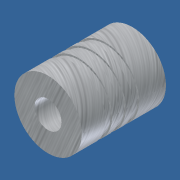
# Autodesk Inventor part: 25772-02
Saved by Autodesk Inventor 2014 (Build 180170000, 170)
## iProperties
Category: stocked
Created: 2011-08-08
Part Number: 25772-02
Document SubType Name: Modeling
Designer: ERF
Density: 2.71 g/cm^3
Description: Z-Axis Flexible Coupler 5mm - 8mm bore
Vendor: Robot Electron
Mass: 18.6653 g
Surface Area: 28.0725 cm^2
Volume: 6.88757 cm^3
Material: Aluminum 6061
Stock Number: ebay
Project: Shapeoko
Appearance: Aluminum (Machined)
Catalog Web Link: http://www.ebay.com/itm/5x5-5x8-5x10-6-35x8-6-35x12-8x8-6x14mm-CNC-Motor-Jaw-Shaft-Coupler-/330796927548
Authority: PER ALLEN @ ROBOT ELECTRON 9-12-13
Title: Flexible Coupler
Author: ERF
Subject: Motion
Comments: Fusion
Autodesk Inventor part; units mm, degrees
ref_plane "YZ Plane" through (0, 0, 0) normal (1, 0, 0) x (0, 1, 0)
ref_plane "XZ Plane" through (0, 0, 0) normal (0, 1, 0) x (-1, 0, 0)
ref_plane "XY Plane" through (0, 0, 0) normal (0, 0, 1) x (1, 0, 0)
sketch "Sketch1" plane through (0, 0, 0) normal (0, 0, 1) x (1, 0, 0)
  circle A0 centre (0, 0) radius 2.5
  circle A1 centre (0, 0) radius 10
  dimension "d0" = 5
  dimension "d1" = 20
  constraints: 2 centre point, 1 coincident
  measures "d0" diameter of A0
  measures "d1" diameter of A1
extrude "Extrusion1" add sketch "Sketch1" along normal blind 25
sketch "Sketch2" plane through (0, 0, 25) normal (0, 0, 1) x (1, 0, 0)
  circle A0 centre (0, 0) radius 2.5 projected
  circle A1 centre (0, 0) radius 10 projected
  circle A2 centre (0, 0) radius 4
  dimension "d4" = 8
  constraints: 1 centre point, 1 coincident
  measures "d4" diameter of A2
extrude "Extrusion2" cut sketch "Sketch2" against normal blind 9.525 contours A2
ref_plane "Work Plane2" through (0, 0, 7.9375) normal (0, 0, -1) x (-1, 0, 0)
sketch "Sketch6" plane through (0, 0, 7.9375) normal (0, 0, -1) x (-1, 0, 0)
  circle A0 centre (0, 0) radius 11
  circle A1 centre (0, 0) radius 9.5
  dimension "d11" = 22
  dimension "d14" = 19
  constraints: 2 centre point, 1 coincident
  measures "d11" diameter of A0
  measures "d14" diameter of A1
extrude "Extrusion5" cut sketch "Sketch6" against normal blind 2
pattern_linear "Rectangular Pattern1" count 3 spacing 4 along (0, 0, 1) of "Extrusion5"
body "Solid1"
